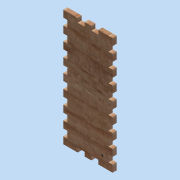
# Autodesk Inventor part: Front_wall
Saved by Autodesk Inventor 2015 (Build 190159000, 159)
## iProperties
Created: 2015-01-31
Part Number: Front_wall
Material: Wood (Birch)
Document SubType Name: Modeling
Designer: Openlab
Density: 0.55 g/cm^3
Appearance: Birch - Natural Polished
Author: Openlab
Autodesk Inventor part; units mm, degrees
ref_plane "YZ Plane" through (0, 0, 0) normal (1, 0, 0) x (0, 1, 0)
ref_plane "XZ Plane" through (0, 0, 0) normal (0, 1, 0) x (-1, 0, 0)
ref_plane "XY Plane" through (0, 0, 0) normal (0, 0, 1) x (1, 0, 0)
sketch "Sketch1" plane through (0, 0, 0) normal (0, 1, 0) x (-1, 0, 0)
  line L0 (0, 0) -> (-3, 0)
  line L1 (-3, 0) -> (-3, -5)
  line L2 (-3, -5) -> (0, -5)
  line L3 (0, -10) -> (-3, -10)
  line L4 (0, -10) -> (0, -5)
  line L5 (-3, -10) -> (-3, -15)
  line L6 (-3, -15) -> (0, -15)
  line L7 (0, -20) -> (-3, -20)
  line L8 (0, -20) -> (0, -15)
  line L9 (-3, -20) -> (-3, -25)
  line L10 (-3, -25) -> (0, -25)
  line L11 (0, -30) -> (-3, -30)
  line L12 (0, -30) -> (0, -25)
  line L13 (-3, -30) -> (-3, -35)
  line L14 (-3, -35) -> (0, -35)
  line L15 (0, -40) -> (-3, -40)
  line L16 (0, -40) -> (0, -35)
  line L17 (-3, -40) -> (-3, -45)
  line L18 (-3, -45) -> (0, -45)
  line L19 (0, -50) -> (-3, -50)
  line L20 (0, -50) -> (0, -45)
  line L21 (-3, -50) -> (-3, -55)
  line L22 (-3, -55) -> (0, -55)
  line L23 (0, -60) -> (-3, -60)
  line L24 (0, -60) -> (0, -55)
  line L25 (-3, -60) -> (-3, -65)
  line L26 (-3, -65) -> (0, -65)
  line L27 (0, -70) -> (-3, -70)
  line L28 (0, -70) -> (0, -65)
  line L29 (-3, -70) -> (-3, -75)
  line L30 (-3, -75) -> (0, -75)
  line L31 (0, -80) -> (-3, -80)
  line L32 (0, -80) -> (0, -75)
  line L33 (0, -20) -> (0, -15)
  line L34 (0, -30) -> (0, -25)
  line L35 (0, -40) -> (0, -35)
  line L36 (0, -50) -> (0, -45)
  line L37 (0, -60) -> (0, -55)
  line L38 (0, -80) -> (0, -75)
  line L39 (0, -70) -> (0, -65)
  line L40 (-3, -80) -> (-3, -85)
  line L41 (-3, -85) -> (0, -85)
  line L42 (30, 0) -> (33, 0)
  line L43 (33, 0) -> (33, -5)
  line L44 (33, -5) -> (30, -5)
  line L45 (30, -10) -> (33, -10)
  line L46 (33, -10) -> (33, -15)
  line L47 (33, -15) -> (30, -15)
  line L48 (30, -20) -> (33, -20)
  line L49 (33, -20) -> (33, -25)
  line L50 (33, -25) -> (30, -25)
  line L51 (30, -30) -> (33, -30)
  line L52 (33, -30) -> (33, -35)
  line L53 (33, -35) -> (30, -35)
  line L54 (30, -40) -> (33, -40)
  line L55 (33, -40) -> (33, -45)
  line L56 (33, -45) -> (30, -45)
  line L57 (30, -50) -> (33, -50)
  line L58 (33, -50) -> (33, -55)
  line L59 (33, -55) -> (30, -55)
  line L60 (30, -60) -> (33, -60)
  line L61 (33, -60) -> (33, -65)
  line L62 (33, -65) -> (30, -65)
  line L63 (30, -70) -> (33, -70)
  line L64 (33, -70) -> (33, -75)
  line L65 (33, -75) -> (30, -75)
  line L66 (30, -80) -> (33, -80)
  line L67 (33, -80) -> (33, -85)
  line L68 (33, -85) -> (30, -85)
  line L69 (30, -75) -> (30, -80)
  line L70 (30, -65) -> (30, -70)
  line L71 (30, -55) -> (30, -60)
  line L72 (30, -45) -> (30, -50)
  line L73 (30, -35) -> (30, -40)
  line L74 (30, -25) -> (30, -30)
  line L75 (30, -5) -> (30, -10)
  line L76 (30, -15) -> (30, -20)
  line L77 (17.5, 0) -> (17.5, -3)
  line L78 (17.5, -3) -> (22.5, -3)
  line L79 (22.5, -3) -> (22.5, 0)
  line L80 (22.5, 0) -> (30, 0)
  line L81 (30, -85) -> (22.5, -85)
  line L82 (7.5, -85) -> (0, -85)
  line L83 (7.5, -85) -> (7.5, -82)
  line L84 (7.5, -82) -> (12.5, -82)
  line L85 (12.5, -82) -> (12.5, -85)
  line L86 (12.5, -85) -> (17.5, -85)
  line L87 (17.5, -85) -> (17.5, -82)
  line L88 (17.5, -82) -> (22.5, -82)
  line L89 (22.5, -82) -> (22.5, -85)
  line L90 (12.5, 0) -> (12.5, -3)
  line L91 (12.5, -3) -> (7.5, -3)
  line L92 (7.5, -3) -> (7.5, 0)
  line L93 (0, 0) -> (7.5, 0)
  line L94 (12.5, 0) -> (17.5, 0)
  point P0 (20, -3)
  dimension "d9" = 10
  dimension "d12" = 10
  dimension "d0" = 30
  dimension "d1" = 85
  dimension "d5" = 5
  dimension "d17" = 3
  dimension "d19" = 3
  dimension "d20" = 7.5
  dimension "d21" = 30
  dimension "d22" = 3
  dimension "d23" = 5
  dimension "d24" = 3
  dimension "d25" = 7.5
  constraints: 190 end point, 41 equal length, 31 perpendicular, 29 collinear, 22 horizontal, 16 point on line, 2 vertical, 1 midpoint
  measures "d0" distance of L68.end L41.end
  measures "d1" distance of L42.start L68.end
  measures "d5" distance between parallel lines of L2 L3
  measures "d17" distance of L0.start L0.end
  measures "d19" distance of L91.end L92.end
  measures "d20" distance from line of L0.start L92
  measures "d21" distance of L42.start L0.start
  measures "d22" distance of L42.start L42.end
  measures "d23" distance of L42.end L43.end
  measures "d24" distance of L88.end L81.end
  measures "d25" distance from line of L41.end L83
extrude "Extrusion1" add sketch "Sketch1" along normal blind 3
equation "\"d17\" = x"
equation "\"d19\" = x"
equation "\"d22\" = x"
equation "\"d24\" = x"
equation "\"x\" = 3"
body "Solid1"
